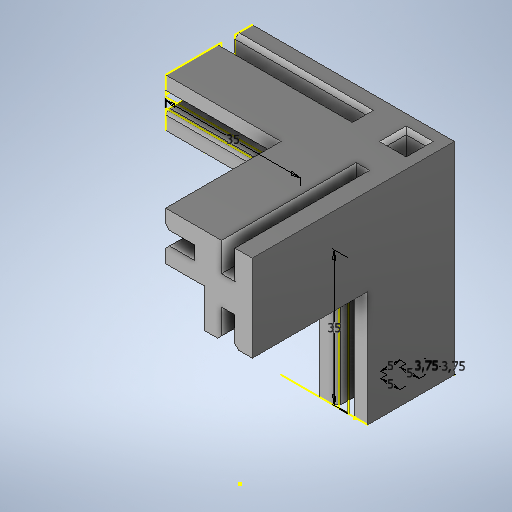
# Autodesk Inventor part: Kątownk Środek Prawy Plexa
Saved by Autodesk Inventor 2025 (Build 290162000, 162)
## iProperties
Created: 2025-07-29
Part Number: Kątownk Środek Prawy Plexa
Material: Ogólny
Document SubType Name: Modeling
Designer: ThePi
Density: 1 g/cm^3
Appearance: Domyślna
d0: 15,000 mm
d6: 1,250 mm
d7: 1,250 mm
d9: 5,000 mm
d10: 5,000 mm
d13: 10,000 mm
d14: 10,000 mm
d15: 5,000 mm
d16: 5,000 mm
d17: 2,500 mm
d18: 5,000 mm
d19: 10,000 mm
d20: 30,000 mm
d21: 0,00 deg
d22: 30,000 mm
d23: 0,00 deg
d24: 30,000 mm
d25: 0,00 deg
d27: 0,00 deg
d28: 5,000 mm
d29: 0,00 deg
d31: 10,000 mm
d34: 0,00 deg
d35: 22,500 mm
d36: 90,00 deg
d37: 10,000 mm
d39: 0,00 deg
d40: 10,000 mm
d41: 0,00 deg
d42: 5,000 mm
d43: 30,000 mm
d44: 2,500 mm
d45: 5,000 mm
d46: 0,00 deg
d47: 30,000 mm
d48: 0,00 deg
d49: 35,000 mm
d50: 35,000 mm
d52: 0,00 deg
d53: 5,000 mm
d55: 0,00 deg
d56: 10,000 mm
d58: 0,00 deg
d77: 0,500 mm
d79: 0,500 mm
d81: 0,500 mm
d83: 0,500 mm
d85: 0,500 mm
d87: 0,500 mm
d92: 5,000 mm
d93: 5,000 mm
d94: 35,000 mm
d95: 0,00 deg
d96: 35,000 mm
d97: 0,00 deg
d105: 4,500 mm
d107: 10,000 mm
d110: 10,000 mm
d111: 10,000 mm
d112: 0,00 deg
d113: 12,000 mm
d114: 0,00 deg
d115: 10,000 mm
d116: 0,00 deg
d124: 5,000 mm
d127: 17,000 mm
d128: 0,00 deg
d129: 3,750 mm
d130: 3,750 mm
d131: 17,000 mm
d132: 0,00 deg
d135: 3,750 mm
d136: 3,750 mm
d137: 5,000 mm
d138: 5,000 mm
d139: 5,000 mm
d140: 17,000 mm
d141: 0,00 deg
d142: 3,750 mm
d143: 3,750 mm
d144: 3,750 mm
d145: 5,000 mm
d146: 5,000 mm
d147: 5,000 mm
d148: 17,000 mm
d149: 0,00 deg
sa_0: 0,400 ul
d156: 2,500 mm
d158: 2,500 mm
d160: 2,500 mm
d162: 2,500 mm
d164: 1,000 mm
d167: 2,500 mm
d173: 1,000 mm
d179: 1,000 mm
d185: 0,500 mm
d187: 0,500 mm
d189: 1,000 mm
d192: 1,000 mm
d30: 10,000 mm
d32: 90,00 deg
Author: ThePi
Autodesk Inventor part; units mm, degrees
ref_plane "YZ Plane" through (0, 0, 0) normal (1, 0, 0) x (0, 1, 0)
ref_plane "XZ Plane" through (0, 0, 0) normal (0, 1, 0) x (-1, 0, 0)
ref_plane "XY Plane" through (0, 0, 0) normal (0, 0, 1) x (1, 0, 0)
sketch "Szkic1" plane through (0, 0, 0) normal (0, 1, 0) x (-1, 0, 0)
  line L0 (0, 0) -> (0, 15)
  line L1 (0, 15) -> (0, 0)
  line L2 (0, 0) -> (15, 0)
  line L3 (3, 10) -> (4.25, 10)
  line L4 (3, 10) -> (1.75, 10)
  line L5 (1.75, 10) -> (1.75, 15)
  line L6 (4.25, 10) -> (4.25, 15)
  line L7 (1.75, 15) -> (-3.25, 15)
  line L8 (4.25, 15) -> (9.25, 15)
  line L9 (-3.25, 15) -> (-3.25, 0)
  line L10 (-3.25, 0) -> (15, 0)
  line L11 (-3.25, 0) -> (11.75, 0)
  line L12 (9.25, 15) -> (9.25, 5)
  line L13 (9.25, 5) -> (19.25, 5)
  line L14 (19.25, 5) -> (19.25, 0)
  line L15 (19.25, 0) -> (14.25, 0)
  line L16 (14.25, 0) -> (14.25, -2.5)
  line L17 (14.25, -2.5) -> (19.25, -2.5)
  line L18 (19.25, -2.5) -> (19.25, -7.5)
  line L19 (19.25, -7.5) -> (9.25, -7.5)
  line L20 (-3.25, 0) -> (-3.25, -7.5)
  line L21 (-3.25, -7.5) -> (9.25, -7.5)
  line L22 (3, 10) -> (3, -1.25)
  line L23 (3, -1.25) -> (14.25, -1.25)
  dimension "d0" = 15
  dimension "d6" = 1.25
  dimension "d7" = 1.25
  dimension "d9" = 5
  dimension "d10" = 5
  dimension "d13" = 10
  dimension "d14" = 10
  dimension "d15" = 5
  dimension "d16" = 5
  dimension "d17" = 2.5
  dimension "d18" = 5
  dimension "d19" = 10
  constraints: 48 end point, 7 perpendicular, 5 point on line, 4 vertical, 2 collinear, 2 horizontal, 1 midpoint, 1 parallel
  measures "d0" distance of L0.start L0.end
  measures "d6" distance of L3.start L3.end
  measures "d7" distance of L3.start L4.end
  measures "d9" distance of L5.end L7.end
  measures "d10" distance of L6.end L8.end
  measures "d13" distance of L8.end L12.end
  measures "d14" distance of L12.end L13.end
  measures "d15" distance of L13.end L14.end
  measures "d16" distance of L14.end L15.end
  measures "d17" distance of L15.end L16.end
  measures "d18" distance of L17.end L18.end
  measures "d19" distance of L18.end L19.end
extrude "Wyciągnięcie proste1" add sketch "Szkic1" along normal blind 30
sketch "Szkic2" plane through (0, 30, 0) normal (0, 1, 0) x (1, 0, 0)
  line L0 (3.25, 7.5) -> (-19.25, 7.5) projected
  line L1 (-19.25, -5) -> (-9.25, -5) projected
  line L2 (-19.25, 7.5) -> (-19.25, -5)
  line L3 (-19.25, -5) -> (-9.25, -5)
  line L4 (-9.25, -5) -> (-9.25, -15) projected
  line L5 (-9.25, -5) -> (-9.25, -15)
  line L6 (-1.75, -15) -> (3.25, -15) projected
  line L7 (-9.25, -15) -> (3.25, -15)
  line L8 (3.25, -15) -> (3.25, 7.5)
  line L9 (3.25, 7.5) -> (-19.25, 7.5)
  point P0 (0, 0)
  constraints: 12 end point, 3 perpendicular, 2 collinear, 1 vertical
extrude "Wyciągnięcie proste2" add sketch "Szkic2" along normal blind 30
sketch "Szkic3" plane through (0, 0, 0) normal (0, -1, 0) x (1, 0, 0)
  point P0 (0, 0)
sketch "Szkic4" plane through (-19.25, 0, -7.5) normal (-1, 0, 0) x (0, 0, 1)
  line L0 (0, 30) -> (12.5, 30)
  line L1 (12.5, 0) -> (12.5, 60) projected
  line L2 (12.5, 30) -> (12.5, 60)
  line L3 (12.5, 60) -> (0, 60)
  line L4 (0, 60) -> (0, 30)
  point P0 (7.5, 0)
  constraints: 8 end point, 2 perpendicular, 1 collinear, 1 midpoint
extrude "Wyciągnięcie proste3" add sketch "Szkic4" along normal blind 30
sketch "Szkic5" plane through (-9.25, 0, 5) normal (-1, 0, 0) x (0, 0, 1)
  line L0 (10, 0) -> (10, 60) projected
  line L1 (10, 30) -> (5, 30) projected
  line L2 (10, 60) -> (10, 30)
  line L3 (10, 30) -> (0, 30)
  line L4 (0, 30) -> (0, 60)
  line L5 (0, 60) -> (10, 60)
  point P0 (-5, 0)
  constraints: 8 end point, 2 perpendicular, 1 collinear, 1 vertical
extrude "Wyciągnięcie proste4" add sketch "Szkic5" along normal up to surface (40 mm away)
sketch "Szkic6" plane through (0, 30, 0) normal (0, -1, 0) x (1, 0, 0)
  line L0 (-14.25, 0) -> (-19.25, 0) projected
  line L1 (-14.25, 0) -> (-49.25, 0)
  line L2 (-49.25, -7.5) -> (-49.25, 15) projected
  line L3 (-49.25, 0) -> (-49.25, -2.5)
  line L4 (-49.25, -2.5) -> (-14.25, -2.5)
  line L5 (-14.25, -2.5) -> (-14.25, 0)
  line L6 (-14.25, 10) -> (-49.25, 10)
  line L7 (-4.25, 10) -> (-1.75, 10) projected
  point P0 (0, 0)
  constraints: 10 end point, 3 point on line, 2 perpendicular, 1 collinear, 1 horizontal, 1 vertical
extrude "Wyciągnięcie proste5" cut sketch "Szkic6" against normal blind 5
sketch "Szkic7" plane through (-1.75, 0, 15) normal (0, 0, 1) x (1, 0, 0)
  line L0 (-7.5, 30) -> (-17.5, 30) projected
  line L1 (-7.5, 30) -> (-17.5, 30)
  line L2 (-7.5, 30) -> (-7.5, 40)
  line L3 (5, 0) -> (5, 60) projected
  line L4 (-7.5, 30) -> (2.5, 30) construction
  line L5 (-7.5, 40) -> (-47.5, 40)
  line L6 (-47.5, 60) -> (-47.5, 30) projected
  line L7 (-47.5, 40) -> (-47.5, 30)
  line L8 (-47.5, 30) -> (-7.5, 30)
  point P0 (1.75, 0)
  dimension "d30" = 10
  dimension "d31" = 10
  dimension "d32" = 90
  constraints: 12 end point, 2 collinear, 2 perpendicular, 1 horizontal, 1 parallel, 1 point on line, 1 vertical
  measures "d30" distance of L0.start L0.end
  measures "d31" distance of L0.start L2.end
  measures "d32" angle of L4 L2
extrude "Wyciągnięcie proste6" cut sketch "Szkic7" against normal up to surface (10 mm away)
sketch "Szkic8" plane through (-49.25, 0, -7.5) normal (-1, 0, 0) x (0, 0, 1)
  point P0 (7.5, 0)
sketch "Szkic9" plane through (0, 0, 0) normal (0, -1, 0) x (1, 0, 0)
  point P0 (0, 0)
sketch "Szkic10" plane through (-49.25, 0, -7.5) normal (-1, 0, 0) x (0, 0, 1)
  line L0 (0, 0) -> (0, 60) projected
  line L1 (0, 30) -> (0, 52.5)
  line L2 (0, 52.5) -> (22.5, 52.5)
  line L3 (22.5, 0) -> (22.5, 60) projected
  line L4 (22.5, 52.5) -> (22.5, 40)
  line L5 (22.5, 40) -> (12.5, 40)
  line L6 (12.5, 40) -> (12.5, 30)
  line L7 (0, 30) -> (5, 30) projected
  line L8 (12.5, 30) -> (0, 30)
  line L9 (22.5, 52.5) -> (22.5, 60)
  line L10 (22.5, 60) -> (0, 60) projected
  line L11 (0, 60) -> (0, 52.5)
  line L12 (22.5, 52.5) -> (0, 52.5)
  point P0 (7.5, 0)
  dimension "d35" = 22.5
  dimension "d36" = 90
  dimension "d37" = 10
  constraints: 18 end point, 4 perpendicular, 3 collinear, 2 point on line, 1 midpoint
  measures "d35" distance of L1.start L1.end
  measures "d36" angle of L1 L2
  measures "d37" distance of L4.end L5.end
sketch "Szkic11" plane through (0, 0, 0) normal (0, -1, 0) x (1, 0, 0)
  point P0 (0, 0)
extrude "Wyciągnięcie proste7" cut sketch "Szkic10" against normal up to surface (52.5 mm away) contours L0 L10 L3 L2
sketch "Szkic12" plane through (-9.25, 0, 15) normal (0, 0, 1) x (1, 0, 0)
  line L0 (12.5, 52.5) -> (-40, 52.5) projected
  line L1 (12.5, 52.5) -> (-10, 52.5)
  line L2 (-10, 30) -> (-40, 30) projected
  line L3 (-10, 52.5) -> (-10, 30)
  line L4 (-10, 30) -> (12.5, 30)
  line L5 (12.5, 0) -> (12.5, 52.5) projected
  line L6 (12.5, 30) -> (12.5, 52.5)
  line L7 (-10, 30) -> (-10, 40)
  line L8 (-40, 40) -> (0, 40) projected
  line L9 (0, 40) -> (0, 30.3734)
  line L10 (0, 0) -> (0, 40) projected
  point P0 (9.25, 0)
  point P1 (0, 30)
  point P2 (0, 40)
  constraints: 12 end point, 3 perpendicular, 3 point on line, 1 parallel
extrude "Wyciągnięcie proste8" add sketch "Szkic12" against normal blind 10 contours L8 L9 L10 L4 L3
sketch "Szkic13" plane through (-9.25, 0, 15) normal (0, 0, 1) x (1, 0, 0)
  line L0 (-40, 52.5) -> (-40, 40) projected
  line L1 (-40, 40) -> (-40, 45)
  line L2 (-40, 45) -> (-10, 45)
  line L3 (-10, 45) -> (-10, 47.5)
  line L4 (-10, 47.5) -> (-40, 47.5)
  line L5 (12.5, 52.5) -> (-40, 52.5) projected
  line L6 (-40, 52.5) -> (-40, 47.5)
  line L7 (-40, 45) -> (-40, 47.5)
  point P0 (9.25, 0)
  dimension "d42" = 5
  dimension "d43" = 30
  dimension "d44" = 2.5
  constraints: 12 end point, 2 collinear, 2 perpendicular, 2 point on line, 1 horizontal
  measures "d42" distance of L0.end L1.end
  measures "d43" distance of L1.end L2.end
  measures "d44" distance of L2.end L3.end
extrude "Wyciągnięcie proste9" cut sketch "Szkic13" against normal blind 5
sketch "Szkic14" plane through (-9.25, 0, 15) normal (0, 0, 1) x (1, 0, 0)
  line L0 (12.5, 0) -> (12.5, 52.5) projected
  line L1 (12.5, 52.5) -> (-10, 52.5)
  line L2 (12.5, 52.5) -> (-40, 52.5) projected
  line L3 (-10, 40) -> (-10, 30) projected
  line L4 (-10, 52.5) -> (-10, 30)
  line L5 (-10, 30) -> (12.5, 30)
  line L6 (12.5, 30) -> (12.5, 52.5)
  point P0 (9.25, 0)
  constraints: 8 end point, 2 perpendicular, 1 point on line, 1 vertical
extrude "Wyciągnięcie proste10" add sketch "Szkic14" along normal blind 30
sketch "Szkic15" plane through (-1.75, 0, 15) normal (0, 0, 1) x (1, 0, 0)
  line L0 (0, 0) -> (0, 30) projected
  line L1 (0, 0) -> (0, 35)
  line L2 (0, 35) -> (0, 0)
  line L3 (-2.5, 0) -> (-2.5, 30) projected
  line L4 (0, 0) -> (-2.5, 0)
  line L5 (5, 0) -> (-17.5, 0) projected
  line L6 (-2.5, 0) -> (-2.5, 35)
  line L7 (-2.5, 35) -> (0, 35)
  line L8 (0, 0) -> (0, 35)
  line L9 (-17.5, 45) -> (-47.5, 45) projected
  line L10 (-47.5, 45) -> (-12.5, 45)
  line L11 (-12.5, 45) -> (-47.5, 45)
  line L12 (-47.5, 47.5) -> (-17.5, 47.5) projected
  line L13 (-47.5, 45) -> (-47.5, 47.5)
  line L14 (-47.5, 47.5) -> (-12.5, 47.5)
  line L15 (-12.5, 47.5) -> (-12.5, 45)
  point P0 (1.75, 0)
  point P1 (-17.5, 47.5)
  dimension "d49" = 35
  dimension "d50" = 35
  constraints: 22 end point, 6 collinear, 2 perpendicular, 2 vertical, 1 parallel
  measures "d49" distance of L0.start L1.end
  measures "d50" distance of L9.end L10.end
extrude "Wyciągnięcie proste11" cut sketch "Szkic15" against normal up to surface (5 mm away)
sketch "Szkic16" plane through (-9.25, 0, 45) normal (0, 0, 1) x (1, 0, 0)
  line L0 (7.5, 0) -> (7.5, 35) projected
  line L1 (7.5, 30) -> (7.5, 35)
  line L2 (5, 35) -> (5, 30) projected
  line L3 (7.5, 35) -> (5, 35)
  line L4 (5, 35) -> (5, 30)
  line L5 (5, 30) -> (7.5, 30)
  line L6 (-10, 40) -> (-10, 45) projected
  line L7 (-10, 45) -> (-5, 45) projected
  line L8 (-10, 45) -> (-5, 45)
  line L9 (-5, 47.5) -> (-10, 47.5) projected
  line L10 (-5, 45) -> (-5, 47.5)
  line L11 (-5, 47.5) -> (-10, 47.5)
  line L12 (-10, 47.5) -> (-10, 45)
  point P0 (9.25, 0)
  dimension "d53" = 5
  constraints: 16 end point, 5 perpendicular, 3 collinear, 1 point on line
  measures "d53" distance of L1.start L0.end
extrude "Wyciągnięcie proste12" cut sketch "Szkic16" against normal up to surface (35 mm away)
sketch "Szkic17" plane through (-9.25, 0, 45) normal (0, 0, 1) x (1, 0, 0)
  line L0 (-10, 30) -> (5, 30) projected
  line L1 (0, 30) -> (0, 40)
  line L2 (-40, 40) -> (-10, 40) projected
  line L3 (0, 40) -> (-10, 40)
  line L4 (-10, 40) -> (-10, 30)
  line L5 (-10, 30) -> (0, 30)
  point P0 (9.25, 0)
  dimension "d56" = 10
  constraints: 8 end point, 3 perpendicular, 1 point on line
  measures "d56" distance of L1.start L1.end
extrude "Wyciągnięcie proste13" cut sketch "Szkic17" against normal up to surface (40 mm away)
thicken "Pogrubienie1" operation cut thickness 0.5 both sides no extend neighbours no toward (-1, 0, 0) faces at (-4.25, 21.6667, 11.6667)
thicken "Pogrubienie2" operation cut thickness 0.5 both sides no extend neighbours no toward (0, 1, 0) faces at (-27.5833, 47.5, 11.6667)
thicken "Pogrubienie3" operation cut thickness 0.5 both sides no extend neighbours no toward (1, 0, 0) faces at (-1.75, 21.6667, 11.6667)
thicken "Pogrubienie4" operation cut thickness 0.5 both sides no extend neighbours no toward (0, -1, 0) faces at (-27.5833, 45, 11.6667)
thicken "Pogrubienie5" operation cut thickness 0.5 both sides no extend neighbours no toward (0, 0, -1) faces at (-15.9167, 21.6667, -2.5)
thicken "Pogrubienie6" operation cut thickness 0.5 both sides no extend neighbours no toward (0, 0, 1) faces at (-27.5833, 33.3333, 0)
sketch "Szkic21" plane through (-49.25, 0, -7.5) normal (-1, 0, 0) x (0, 0, 1)
  line L0 (4.5, 35) -> (8, 35) projected
  line L1 (4.5, 35) -> (4.5, 52.5)
  line L2 (22.5, 52.5) -> (0, 52.5) projected
  line L3 (8, 0) -> (8, 35) projected
  line L4 (8, 35) -> (8, 52.5)
  line L5 (8, 52.5) -> (4.5, 52.5)
  line L6 (4.5, 52.5) -> (4.5, 47.5)
  line L7 (4.5, 47.5) -> (8, 47.5)
  point P0 (7.5, 0)
  dimension "d92" = 5
  constraints: 10 end point, 3 point on line, 2 perpendicular, 2 vertical
  measures "d92" distance of L1.end L6.end
sketch "Szkic22" plane through (-9.25, 0, 45) normal (0, 0, 1) x (1, 0, 0)
  point P0 (9.25, 0)
sketch "Szkic23" plane through (-9.25, 0, 45) normal (0, 0, 1) x (1, 0, 0)
  line L0 (4.5, 35) -> (8, 35) projected
  line L1 (4.5, 35) -> (4.5, 52.5)
  line L2 (12.5, 52.5) -> (-10, 52.5) projected
  line L3 (8, 35) -> (8, 52.5)
  line L4 (8, 52.5) -> (4.5, 52.5)
  line L5 (4.5, 52.5) -> (4.5, 47.5)
  line L6 (4.5, 47.5) -> (8, 47.5)
  point P0 (9.25, 0)
  dimension "d93" = 5
  constraints: 10 end point, 3 point on line, 2 vertical, 1 collinear, 1 perpendicular
  measures "d93" distance of L1.end L5.end
extrude "Wyciągnięcie proste17" cut sketch "Szkic21" against normal blind 35 contours L1 L2 L4 L7
extrude "Wyciągnięcie proste18" cut sketch "Szkic23" against normal blind 35 contours L1 L2 L3 L6
sketch "Szkic25" plane through (-49.25, 52.5, -7.5) normal (0, 1, 0) x (1, 0, 0)
  line L0 (0, -8) -> (0, -4.5) projected
  line L1 (0, -4.5) -> (0, -8)
  line L2 (0, -8) -> (35, -8)
  line L3 (35, -8) -> (35, -4.5)
  line L4 (35, -4.5) -> (0, -4.5)
  point P0 (49.25, -7.5)
  constraints: 8 end point, 3 perpendicular, 1 collinear
sketch "Szkic26" plane through (-49.25, 52.5, -7.5) normal (0, 1, 0) x (1, 0, 0)
  line L0 (44.5, -17.5) -> (44.5, -22.5) projected
  line L1 (44.5, -17.5) -> (52.5, -17.5)
  line L2 (52.5, 0) -> (52.5, -52.5) projected
  line L3 (44.5, -17.5) -> (40, -17.5)
  line L4 (35, -8) -> (35, -4.5) projected
  line L5 (35, -12.5) -> (40, -12.5)
  line L6 (40, -12.5) -> (40, -17.5)
  line L7 (52.5, -22.5) -> (48, -22.5) projected
  line L8 (48, -17.5) -> (48, -22.5)
  line L9 (48, -22.5) -> (48, -12.5)
  line L10 (48, -12.5) -> (52.5, -12.5)
  line L11 (52.5, -22.5) -> (52.5, -12.5)
  line L12 (30, -8) -> (35, -8) projected
  line L13 (35, -8) -> (30, -8)
  line L14 (30, -22.5) -> (0, -22.5) projected
  line L15 (30, -22.5) -> (30, -12.5)
  line L16 (30, -12.5) -> (52.5, -12.5)
  line L17 (30, -12.5) -> (40, -12.5)
  line L18 (40, -12.5) -> (40, 0)
  line L19 (40, -52.5) -> (40, -12.5) projected
  line L20 (40, -12.5) -> (52.5, -12.5)
  line L21 (40, 0) -> (40, -12.5)
  line L22 (40, -12.5) -> (0, -12.5)
  line L23 (0, -12.5) -> (0, -8)
  line L24 (0, -8) -> (35, -8)
  line L25 (35, -8) -> (35, -4.5)
  line L26 (35, -4.5) -> (30, -4.5) projected
  line L27 (30, -4.5) -> (0, -4.5) projected
  line L28 (35, -4.5) -> (0, -4.5)
  line L29 (0, -4.5) -> (0, 0)
  line L30 (0, 0) -> (40, 0)
  line L31 (40, 0) -> (52.5, 0)
  line L32 (52.5, 0) -> (52.5, -12.5)
  line L33 (44.5, -17.5) -> (48, -17.5) projected
  line L34 (40, -12.5) -> (52.5, -12.5)
  line L35 (52.5, -52.5) -> (52.5, -12.5)
  line L36 (52.5, -52.5) -> (30, -52.5) projected
  line L37 (52.5, -52.5) -> (48, -52.5)
  line L38 (48, -17.5) -> (48, -52.5) projected
  line L39 (48, -52.5) -> (48, -17.5)
  line L40 (48, -17.5) -> (44.5, -17.5) projected
  line L41 (48, -17.5) -> (44.5, -17.5)
  line L42 (44.5, -52.5) -> (44.5, -17.5) projected
  line L43 (44.5, -17.5) -> (44.5, -52.5)
  line L44 (44.5, -52.5) -> (40, -52.5)
  line L45 (40, -52.5) -> (40, -12.5)
  point P0 (49.25, -7.5)
  dimension "d105" = 4.5
  dimension "d107" = 10
  dimension "d110" = 10
  constraints: 64 end point, 10 collinear, 9 point on line, 7 perpendicular, 3 horizontal, 1 vertical
  measures "d105" distance of L0.start L3.end
  measures "d107" distance of L7.end L9.end
  measures "d110" distance of L14.start L15.end
extrude "Wyciągnięcie proste20" [suppressed]
sketch "Szkic27" plane through (-4.75, 47.5, 45) normal (0, 1, 0) x (1, 0, 0)
  line L0 (3.5, 35) -> (0, 35)
  line L1 (-14.5, 48) -> (-44.5, 48) projected
  line L2 (-44.5, 48) -> (-44.5, 44.5) projected
  line L3 (-44.5, 48) -> (-44.5, 44.5)
  line L4 (-9.5, 48) -> (-9.5, 44.5) projected
  line L5 (-44.5, 44.5) -> (-9.5, 44.5)
  line L6 (-9.5, 44.5) -> (-9.5, 48)
  line L7 (-9.5, 48) -> (-44.5, 48.1482)
  line L8 (3.5, 0) -> (3.5, 35) projected
  line L9 (3.5, 0) -> (0, 0) projected
  line L10 (3.5, 0) -> (0, 0)
  line L11 (0, 0) -> (0, 35)
  line L12 (0, 35) -> (3.5, 35)
  line L13 (3.5, 0) -> (3.5, 35)
  point P0 (4.75, 45)
  constraints: 18 end point, 4 perpendicular, 3 collinear, 1 point on line
extrude "Wyciągnięcie proste21" [suppressed]
extrude "Wyciągnięcie proste22" [suppressed]
sketch "Szkic29" plane through (-49.25, 62.5, -7.5) normal (0, 1, 0) x (1, 0, 0)
  line L0 (52.5, 0) -> (0, 0) projected
  line L1 (52.5, 0) -> (48.75, 0)
  line L2 (48.75, 0) -> (52.5, 0)
  line L3 (52.5, 0) -> (48.75, 0)
  line L4 (48.75, -3.75) -> (43.75, -3.75)
  line L5 (43.75, -3.75) -> (43.75, -8.75)
  line L6 (43.75, -8.75) -> (48.75, -8.75)
  line L7 (48.75, -8.75) -> (48.75, -3.75)
  point P0 (49.25, -7.5)
  dimension "d124" = 5
  constraints: 14 end point, 2 collinear, 1 perpendicular, 1 point on line
  measures "d124" distance of L4.start L4.end
extrude "Wyciągnięcie proste24" [suppressed]
sketch "Szkic30" plane through (0, 0, 0) normal (0, -1, 0) x (1, 0, 0)
  line L0 (3.25, -7.5) -> (-49.25, -7.5) projected
  line L1 (3.25, -7.5) -> (-0.5, -7.5)
  line L2 (-0.5, -7.5) -> (-0.5, -3.75)
  line L3 (-0.5, 1.25) -> (-5.5, 1.25) projected
  line L4 (-0.5, 1.25) -> (-0.5, -3.75)
  line L5 (-5.5, 1.25) -> (-5.5, -3.75) projected
  line L6 (-5.5, 1.2502) -> (-5.5, -3.75)
  line L7 (-5.5, -3.75) -> (-0.5, -3.75)
  point P0 (0, 0)
  dimension "d129" = 3.75
  dimension "d130" = 3.75
  constraints: 10 end point, 1 collinear, 1 perpendicular, 1 point on line
  measures "d129" distance of L0.start L1.end
  measures "d130" distance of L1.end L2.end
extrude "Wyciągnięcie proste25" [suppressed]
sketch "Szkic31" plane through (-49.25, 52.5, -7.5) normal (0, 1, 0) x (1, 0, 0)
  line L0 (0, 0) -> (52.5, 0) projected
  line L1 (52.5, 0) -> (48.75, 0)
  line L2 (48.75, 0) -> (48.75, -3.75)
  line L3 (52.5, 0) -> (48.75, 0)
  line L4 (48.75, 0) -> (48.75, -3.75)
  line L5 (48.75, -3.75) -> (43.75, -3.75)
  line L6 (43.75, -3.75) -> (43.75, -8.75)
  line L7 (43.75, -8.75) -> (48.75, -8.75)
  line L8 (48.75, -8.75) -> (48.75, -3.75)
  point P0 (49.25, -7.5)
  dimension "d135" = 3.75
  dimension "d136" = 3.75
  dimension "d137" = 5
  dimension "d138" = 5
  dimension "d139" = 5
  constraints: 16 end point, 3 perpendicular, 2 collinear, 2 point on line
  measures "d135" distance of L0.end L1.end
  measures "d136" distance of L1.end L2.end
  measures "d137" distance of L2.end L5.end
  measures "d138" distance of L5.end L6.end
  measures "d139" distance of L6.end L7.end
extrude "Wyciągnięcie proste26" cut sketch "Szkic31" against normal blind 17
sketch "Szkic32" plane through (0, 0, 0) normal (0, -1, 0) x (1, 0, 0)
  line L0 (-49.25, -7.5) -> (3.25, -7.5) projected
  line L1 (3.25, -7.5) -> (-0.5, -7.5)
  line L2 (-0.5, -7.5) -> (-4.25, -7.5)
  line L3 (-4.25, -7.5) -> (-0.5, -7.5)
  line L4 (-0.5, -7.5) -> (-0.5, -3.75)
  line L5 (-0.5, -3.75) -> (-5.5, -3.75)
  line L6 (-5.5, -3.75) -> (-5.5, 1.25)
  line L7 (-5.5, 1.25) -> (-0.5, 1.25)
  line L8 (-0.5, 1.25) -> (-0.5, -3.75)
  point P0 (0, 0)
  dimension "d142" = 3.75
  dimension "d143" = 3.75
  dimension "d144" = 3.75
  dimension "d145" = 5
  dimension "d146" = 5
  dimension "d147" = 5
  constraints: 16 end point, 3 perpendicular, 3 point on line, 2 collinear
  measures "d142" distance of L0.end L1.end
  measures "d143" distance of L1.end L2.end
  measures "d144" distance of L1.end L4.end
  measures "d145" distance of L4.end L5.end
  measures "d146" distance of L5.end L6.end
  measures "d147" distance of L6.end L7.end
extrude "Wyciągnięcie proste27" cut sketch "Szkic32" against normal blind 17
sketch "Szkic33" plane through (-49.25, 0, -7.5) normal (-1, 0, 0) x (0, 0, 1)
  line L0 (4.5, 30) -> (4.5, 35) projected
  line L1 (4.5, 35) -> (8, 35) projected
  line L2 (8, 35) -> (8, 30) projected
  line L3 (8, 30) -> (12.5, 30) projected
  line L4 (12.5, 30) -> (12.5, 40) projected
  line L5 (12.5, 40) -> (22.5, 40) projected
  line L6 (22.5, 44.5) -> (22.5, 40) projected
  line L7 (22.5, 44.5) -> (17.5, 44.5) projected
  line L8 (17.5, 44.5) -> (17.5, 48) projected
  line L9 (17.5, 48) -> (22.5, 48) projected
  line L10 (22.5, 52.5) -> (22.5, 48) projected
  line L11 (4.5, 52.5) -> (0, 52.5) projected
  line L12 (8, 52.5) -> (8, 47.5) projected
  line L13 (8, 47.5) -> (4.5, 47.5) projected
  line L14 (4.5, 47.5) -> (4.5, 52.5) projected
  line L15 (22.5, 52.5) -> (8, 52.5) projected
  line L16 (0, 52.5) -> (0, 30) projected
  line L17 (0, 30) -> (4.5, 30) projected
  point P0 (7.5, 0)
thicken "Pogrubienie8" operation cut thickness 2.5 both sides no extend neighbours no toward (0, 0, -1) faces at (-3.5833, 23.3333, 10) (-3.5833, 35, 21.6667)
thicken "Pogrubienie9" operation cut thickness 2.5 both sides no extend neighbours no toward (1, 0, 0) faces at (-14.25, 11.6667, -0.6667) (-25.9167, 35, -0.6667)
thicken "Pogrubienie10" operation cut thickness 2.5 both sides no extend neighbours no toward (0, -1, 0) faces at (-37.5833, 47.5, -1.8333)
thicken "Pogrubienie11" operation cut thickness 2.5 both sides no extend neighbours no toward (1, 0, 0) faces at (-14.25, 45.6667, 21.6667) (-25.9167, 46.8333, 10)
chamfer "Faza6" distance 1 angle 45 8 edges at (-3, 0, 1.25) (-0.5, 0, -1.25) (-3, 0, -3.75) (-5.5, 0, -1.25) (-5.5, 52.5, -1.25) (-3, 52.5, -3.75) (-0.5, 52.5, -1.25) (-3, 52.5, 1.25)
thicken "Pogrubienie12" operation cut thickness 2.5 both sides no extend neighbours no toward (0, -1, 0) faces at (-3.5833, 47.5, 33.3333)
chamfer "Faza7" distance 1 angle 45 4 edges at (-19.25, 48, 30) (-19.25, 44.5, 30) (-34.25, 48, 15) (-34.25, 44.5, 15)
chamfer "Faza9" distance 1 angle 45 4 edges at (-4.75, 30, 30) (-1.25, 30, 30) (-1.25, 15, 15) (-4.75, 15, 15)
thicken "Pogrubienie15" operation add thickness 0.5 both sides no extend neighbours no toward (0, 0, -1) faces at (-14.25, 22.5, 0.5)
thicken "Pogrubienie16" operation add thickness 0.5 both sides no extend neighbours no toward (0, 0, 1) faces at (-14.25, 22.5, -3)
chamfer "Faza11" [suppressed]
chamfer "Faza12" distance 1 angle 45 2 edges at (-31.75, 52.5, 0.5) (-31.75, 52.5, -3)
